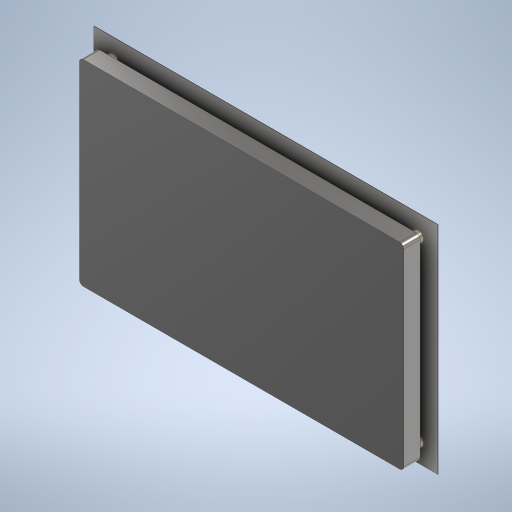
# Autodesk Inventor part: monitor-stand
Saved by Autodesk Inventor 2023 (Build 270158030, 158C)
## iProperties
Created: 2024-02-27
Part Number: monitor-stand
Material: Generic
Document SubType Name: Modeling
Designer: Imogen Heard
Density: 1 g/cm^3
Appearance: Expanded Metal 01
Author: Imogen Heard
Autodesk Inventor part; units mm, degrees
ref_plane "YZ Plane" through (0, 0, 0) normal (1, 0, 0) x (0, 1, 0)
ref_plane "XZ Plane" through (0, 0, 0) normal (0, 1, 0) x (-1, 0, 0)
ref_plane "XY Plane" through (0, 0, 0) normal (0, 0, 1) x (1, 0, 0)
sketch "Sketch1" plane through (0, 0, 0) normal (0, 0, 1) x (1, 0, 0)
  line L0 (-82.5, 50) -> (82.5, 50)
  line L1 (82.5, 50) -> (82.5, -50)
  line L2 (82.5, -50) -> (-82.5, -50)
  line L3 (-82.5, -50) -> (-82.5, 50)
  point P0 (0, 0)
  dimension "d0" = 165
  dimension "d1" = 100
  dimension "d2" = 82.5
  dimension "d3" = 50
  constraints: 8 end point, 2 parallel, 1 horizontal, 1 perpendicular
  measures "d0" distance between parallel lines of L1 L3
  measures "d1" distance between parallel lines of L2 L0
  measures "d2" horizontal distance of L2.end point (0, 0)
  measures "d3" distance from line of L2 point (0, 0)
extrude "Extrusion1" add sketch "Sketch1" along normal blind 8.36
sketch "Sketch2" plane through (0, 0, 0) normal (0, 0, -1) x (-1, 0, 0)
  circle A0 centre (-77.5, 45) radius 2.75
  circle A1 centre (77.5, 45) radius 2.75
  circle A2 centre (77.5, -45) radius 2.75
  circle A3 centre (-77.5, -45) radius 2.75
  line L0 (-82.5, 50) -> (82.5, 50) projected
  line L1 (-82.5, -50) -> (-82.5, 50) projected
  line L2 (82.5, -50) -> (-82.5, -50) projected
  line L3 (82.5, 50) -> (82.5, -50) projected
  point P0 (0, 0)
  dimension "d6" = 5.5
  dimension "d7" = 5
  dimension "d8" = 5
  dimension "d9" = 5
  dimension "d10" = 5
  constraints: 4 centre point, 3 equal radius, 2 horizontal alignment, 2 vertical alignment
  measures "d6" diameter of A3
  measures "d7" distance from line of L0 A0.centre
  measures "d8" distance from line of L1 A0.centre
  measures "d9" distance from line of L2 A3.centre
  measures "d10" distance from line of L3 A2.centre
extrude "Extrusion2" add sketch "Sketch2" along normal blind 4 contours A0 | A1 | A2 | A3
hole "Hole1" at (-77.5, -45, -4) direction (0, 0, 1) diameter 2.013 depth 4 tip angle 118 start extended yes countersink diameter 4 countersink angle 90 thread size "M2.5x0.45" class "6H" standard "ISO Metric profile"
hole "Hole2" at (77.5, 45, -4) direction (0, 0, 1) diameter 2.013 depth 4 tip angle 118 start extended yes countersink diameter 4 countersink angle 90 thread size "M2.5x0.45" class "6H" standard "ISO Metric profile"
hole "Hole3" at (77.5, -45, -4) direction (0, 0, 1) diameter 2.013 depth 4 tip angle 118 start extended yes countersink diameter 4 countersink angle 90 thread size "M2.5x0.45" class "6H" standard "ISO Metric profile"
hole "Hole4" at (-77.5, 45, -4) direction (0, 0, 1) diameter 2.013 depth 4 tip angle 118 start extended yes countersink diameter 4 countersink angle 90 thread size "M2.5x0.45" class "6H" standard "ISO Metric profile"
fillet "Fillet1" radius 2 4 edges at (82.5, 50, 4.18) (-82.5, 50, 4.18) (82.5, -50, 4.18) (-82.5, -50, 4.18)
sketch "Sketch4" plane through (0, 0, 0) normal (0, 0, -1) x (-1, 0, 0)
  line L0 (81.5, 35) -> (73.35, 35)
  line L1 (73.35, 35) -> (73.35, 23)
  line L2 (73.35, 23) -> (81.5, 23)
  line L3 (81.5, 23) -> (81.5, 35)
  line L4 (-80.5, 50) -> (80.5, 50) projected
  line L5 (82.5, 48) -> (82.5, -48) projected
  point P0 (0, 0)
  dimension "d54" = 15
  dimension "d55" = 12
  dimension "d56" = 9.15
  dimension "d57" = 1
  constraints: 8 end point, 2 parallel, 1 horizontal, 1 perpendicular
  measures "d54" distance between parallel lines of L0 L4
  measures "d55" distance between parallel lines of L2 L0
  measures "d56" distance between parallel lines of L5 L1
  measures "d57" distance between parallel lines of L5 L3
extrude "Extrusion3" add sketch "Sketch4" along normal blind 3
fillet "Fillet2" radius 6 2 edges at (-81.5, 35, -1.5) (-81.5, 23, -1.5)
sketch "Sketch5" plane through (0, 0, 0) normal (0, 0, -1) x (-1, 0, 0)
  arc A0 (77.425, 21.5) -> (77.425, 36.5) centre (77.425, 29) ccw
  line L0 (73.35, 35) -> (73.35, 23) projected
  line L1 (73.35, 23) -> (75.5, 23) projected
  line L2 (75.5, 35) -> (73.35, 35) projected
  line L3 (81.5, 35) -> (73.35, 35) projected
  line L4 (77.425, 36.5) -> (77.425, 21.5)
  arc A1 (75.5, 23) -> (75.5, 35) centre (75.5, 29) ccw projected
  point P0 (0, 0)
  point P1 (77.425, 35)
  point P2 (77.425, 35)
  point P3 (77.425, 23)
  point P4 (77.425, 34.6828)
  point P5 (77.425, 23.3172)
  point P6 (77.425, 35)
  dimension "d60" = 15
  dimension "d61" = 12
  dimension "d62" = 6
  dimension "d64" = 4.075
  constraints: 2 end point, 2 point on circle, 1 centre point, 1 midpoint
  measures "d60" diameter of A0
  measures "d61" distance from line of point (77.425, 35) L1
  measures "d62" distance from line of L1 A0.centre
  measures "d64" distance from line of L0 A0.centre
extrude "Extrusion4" add sketch "Sketch5" along normal blind 2.7 contours L4 A1 A0 | L4 A1
sketch "Sketch6" plane through (-82.5, -48, 8.36) normal (-1, 0, 0) x (0, 0, 1)
  line L0 (-14.66, 18.5) -> (-10.47, 18.5)
  line L1 (-10.47, 33.5) -> (-14.66, 33.5)
  line L2 (-14.66, 33.5) -> (-14.66, 18.5)
  line L3 (-10.47, 20) -> (-9.06, 21)
  line L4 (-9.06, 21) -> (-9.06, 31)
  line L5 (-8.36, 0) -> (-8.36, 96) projected
  line L6 (-9.06, 31) -> (-10.47, 32)
  line L7 (-10.47, 33) -> (-8.36, 33)
  line L8 (-8.36, 33) -> (-8.36, 33.5)
  line L9 (-8.36, 33.5) -> (-10.47, 33.5)
  line L10 (-10.47, 18.5) -> (-8.36, 18.5)
  line L11 (-8.36, 18.5) -> (-8.36, 19)
  line L12 (-8.36, 19) -> (-10.47, 19)
  line L13 (-8.36, -2) -> (0, -2) projected
  line L14 (-10.47, 19) -> (-10.47, 20)
  line L15 (-10.47, 32) -> (-10.47, 33)
  line L16 (-10.92, 33.05) -> (-10.92, 31.7675)
  line L17 (-10.92, 31.7675) -> (-9.51, 30.7675)
  line L18 (-9.51, 30.7675) -> (-9.51, 21.2325)
  line L19 (-9.51, 21.2325) -> (-10.92, 20.2325)
  line L20 (-10.92, 20.2325) -> (-10.92, 18.95)
  line L21 (-10.92, 18.95) -> (-14.21, 18.95)
  line L22 (-14.21, 18.95) -> (-14.21, 33.05)
  line L23 (-14.21, 33.05) -> (-10.92, 33.05)
  point P0 (-8.36, 48)
  point P1 (-12.565, 33.05)
  point P2 (-10.47, 32.5)
  point P3 (-10.47, 19.5)
  point P4 (-8.36, 18.5)
  point P5 (-10.47, 33.5)
  dimension "d68" = 0.5
  dimension "d69" = 0.5
  dimension "d70" = 15
  dimension "d71" = 6.3
  dimension "d73" = 0.7
  dimension "d74" = 1.5
  dimension "d75" = 1.5
  dimension "d76" = 20.5
  dimension "d77" = 2.5
  dimension "d78" = 2.5
  dimension "d79" = 2.11
  dimension "d80" = 0.45
  dimension "d81" = 0.45
  dimension "d82" = 0.45
  dimension "d83" = 0.45
  dimension "d84" = 0.45
  dimension "d85" = 0.45
  constraints: 44 end point, 9 parallel, 6 perpendicular, 3 horizontal, 3 midpoint, 2 point on line, 1 coincident, 1 vertical alignment, 2 other
  measures "d68" distance between parallel lines of L9 L7
  measures "d69" distance between parallel lines of L12 L10
  measures "d70" distance between parallel lines of L1 L0
  measures "d71" distance between parallel lines of L5 L2
  measures "d73" distance between parallel lines of L5 L4
  measures "d74" distance from line of L1 L6.end
  measures "d75" distance from line of L0 L3.start
  measures "d76" distance between parallel lines of L13 L0
  measures "d77" distance from line of L1 L4.end
  measures "d78" distance from line of L0 L3.end
  measures "d79" distance between parallel lines of L5 L15
  measures "d80" distance between parallel lines of L2 L22
  measures "d81" distance from line of L1 point (-12.565, 33.05)
  measures "d82" distance between parallel lines of L4 L18
  measures "d83" distance from line of point (-10.47, 32.5) L16
  measures "d84" distance between parallel lines of L0 L21
  measures "d85" distance from line of point (-10.47, 19.5) L20
extrude "Extrusion5" add sketch "Sketch6" along normal blind 0.4 and the other way blind 12 contours L2 L1 L9 L5 L7 L15 L6 L4 L3 L14 L12 L10 L0
fillet "Fillet3" radius 0.5 6 edges at (-76.7, -14.5, -6.3) (-76.7, -29.5, -6.3) (-76.7, -27.7675, -2.56) (-76.7, -16.2325, -2.56) (-76.7, -17, -0.7) (-76.7, -27, -0.7)
fillet "Fillet4" radius 0.2 8 edges at (-76.7, -29.05, -5.85) (-76.7, -14.95, -5.85) (-76.7, -29.05, -2.56) (-76.7, -26.7675, -1.15) (-76.7, -17.2325, -1.15) (-76.7, -14.95, -2.56) (-76.7, -16, -2.11) (-76.7, -28, -2.11)
sketch "Sketch7" plane through (-70.5, -48, 8.36) normal (-1, 0, 0) x (0, 0, -1)
  arc A0 (9.2708, -20.8505) -> (9.06, -21.2584) centre (9.56, -21.2584) ccw projected
  line L0 (10.3857, -20.0598) -> (9.2708, -20.8505) projected
  arc A1 (10.3857, -20.0598) -> (10.47, -19.8967) centre (10.27, -19.8967) ccw projected
  line L1 (10.47, -19) -> (10.47, -19.8967) projected
  line L2 (8.36, -19) -> (10.47, -19) projected
  line L3 (14.16, -18.5) -> (8.36, -18.5) projected
  arc A2 (14.66, -19) -> (14.16, -18.5) centre (14.16, -19) ccw projected
  line L4 (14.66, -33) -> (14.66, -19) projected
  arc A3 (14.16, -33.5) -> (14.66, -33) centre (14.16, -33) ccw projected
  line L5 (8.36, -33.5) -> (14.16, -33.5) projected
  line L6 (10.47, -33) -> (8.36, -33) projected
  line L7 (10.47, -32.1033) -> (10.47, -33) projected
  arc A4 (10.47, -32.1033) -> (10.3857, -31.9402) centre (10.27, -32.1033) ccw projected
  line L8 (9.2708, -31.1495) -> (10.3857, -31.9402) projected
  arc A5 (9.06, -30.7416) -> (9.2708, -31.1495) centre (9.56, -30.7416) ccw projected
  line L9 (9.06, -21.2584) -> (9.06, -30.7416) projected
  arc A6 (10.92, -32.0258) -> (10.7092, -31.618) centre (10.42, -32.0258) ccw projected
  line L10 (10.92, -32.85) -> (10.92, -32.0258) projected
  arc A7 (10.92, -32.85) -> (11.12, -33.05) centre (11.12, -32.85) ccw projected
  line L11 (14.01, -33.05) -> (11.12, -33.05) projected
  arc A8 (14.01, -33.05) -> (14.21, -32.85) centre (14.01, -32.85) ccw projected
  line L12 (14.21, -19.15) -> (14.21, -32.85) projected
  arc A9 (14.21, -19.15) -> (14.01, -18.95) centre (14.01, -19.15) ccw projected
  line L13 (11.12, -18.95) -> (14.01, -18.95) projected
  arc A10 (11.12, -18.95) -> (10.92, -19.15) centre (11.12, -19.15) ccw projected
  line L14 (10.92, -19.9742) -> (10.92, -19.15) projected
  arc A11 (10.7092, -20.382) -> (10.92, -19.9742) centre (10.42, -19.9742) ccw projected
  line L15 (9.5943, -21.1727) -> (10.7092, -20.382) projected
  arc A12 (9.5943, -21.1727) -> (9.51, -21.3359) centre (9.71, -21.3359) ccw projected
  line L16 (9.51, -30.6641) -> (9.51, -21.3359) projected
  arc A13 (9.51, -30.6641) -> (9.5943, -30.8273) centre (9.71, -30.6641) ccw projected
  line L17 (10.7092, -31.618) -> (9.5943, -30.8273) projected
  line L18 (8.36, -33) -> (8.36, -33.5) projected
  line L19 (8.36, -18.5) -> (8.36, -19) projected
  point P0 (8.36, -48)
extrude "Extrusion6" add sketch "Sketch7" along normal blind 4.5 contours A6 L17 A13 L16 A12 L15 A11 L14 A10 L13 A9 L12 A8 L11 A7 L10
sketch "Sketch8" plane through (-82.5, -48, 8.36) normal (-1, 0, 0) x (0, 0, 1)
  line L0 (-10.06, 42.6) -> (-10.06, 48.5) construction
  line L1 (-8.46, 42.6) -> (-8.46, 48.5)
  line L2 (-11.66, 48.5) -> (-11.66, 42.6)
  arc A0 (-11.66, 42.6) -> (-8.46, 42.6) centre (-10.06, 42.6) ccw
  arc A1 (-8.46, 48.5) -> (-11.66, 48.5) centre (-10.06, 48.5) ccw
  line L3 (-8.36, 71.4778) -> (-8.36, 33.5) projected
  line L4 (-11.31, 42.6) -> (-11.31, 48.5)
  arc A2 (-8.81, 48.5) -> (-11.31, 48.5) centre (-10.06, 48.5) ccw
  line L5 (-8.81, 48.5) -> (-8.81, 42.6)
  arc A3 (-11.31, 42.6) -> (-8.81, 42.6) centre (-10.06, 42.6) ccw
  point P0 (-8.36, 48)
  point P1 (-10.06, 45.55)
  point P2 (-10.06, 50.1)
  point P3 (-10.06, 41)
  point P4 (-8.36, -2)
  dimension "d94" = 9.1
  dimension "d95" = 3.2
  dimension "d96" = 0.1
  dimension "d97" = 43
  dimension "d98" = 0.35
  constraints: 12 end point, 10 point on circle, 4 centre point, 4 tangent, 2 parallel, 1 midpoint, 1 vertical, 3 other
  measures "d94" distance of point (-10.06, 50.1) point (-10.06, 41)
  measures "d95" distance between parallel lines of L1 L2
  measures "d96" distance between parallel lines of L3 L1
  measures "d97" vertical distance of point (-8.36, -2) point (-10.06, 41)
  measures "d98" distance between parallel lines of L2 L4
extrude "Extrusion7" add sketch "Sketch8" against normal blind 7.5
sketch "Sketch9" plane through (-75, -48, 8.36) normal (1, 0, 0) x (0, 0, -1)
  arc A0 (11.66, 48.5) -> (8.46, 48.5) centre (10.06, 48.5) ccw projected
  line L0 (8.46, 48.5) -> (8.46, 42.6) projected
  arc A1 (8.46, 42.6) -> (11.66, 42.6) centre (10.06, 42.6) ccw projected
  line L1 (11.66, 42.6) -> (11.66, 48.5) projected
  line L2 (8.81, 42.6) -> (8.81, 48.5) projected
  arc A2 (11.31, 48.5) -> (8.81, 48.5) centre (10.06, 48.5) ccw projected
  line L3 (11.31, 48.5) -> (11.31, 42.6) projected
  arc A3 (8.81, 42.6) -> (11.31, 42.6) centre (10.06, 42.6) ccw projected
  point P0 (8.36, 48)
extrude "Extrusion8" add sketch "Sketch9" against normal blind 2 contours L2 A2 L3 A3
sketch "Sketch10" plane through (-82.5, -48, 8.36) normal (-1, 0, 0) x (0, 0, 1)
  circle A0 centre (-10.91, 59) radius 2.45
  circle A1 centre (-10.91, 59) radius 1.72
  line L0 (-8.36, 71.4778) -> (-8.36, 33.5) projected
  line L1 (0, 98) -> (-8.36, 98) projected
  point P0 (-8.36, 48)
  dimension "d103" = 4.9
  dimension "d104" = 0.73
  dimension "d105" = 2.55
  dimension "d106" = 39
  constraints: 2 centre point, 1 concentric
  measures "d103" diameter of A0
  measures "d104" radial gap between concentric circles of A0 A1
  measures "d105" distance from line of L0 A0.centre
  measures "d106" distance from line of L1 A0.centre
extrude "Extrusion9" add sketch "Sketch10" against normal blind 14
sketch "Sketch11" plane through (-68.5, 11, -2.55) normal (1, 0, 0) x (0, 0, -1)
  line L0 (-2.55, 12.4778) -> (-2.55, -25.5) projected
  line L1 (2.45, 3.175) -> (-2.55, 3.175)
  line L2 (-2.55, 3.175) -> (-2.55, -3.175)
  line L3 (-2.55, -3.175) -> (2.45, -3.175)
  line L4 (2.45, -3.175) -> (2.45, 3.175)
  circle A0 centre (0, 0) radius 1.72 projected
  point P0 (-2.55, -11)
  point P1 (-2.55, 3.175)
  dimension "d109" = 6.35
  dimension "d110" = 3.175
  dimension "d111" = 5
  constraints: 8 end point, 2 parallel, 1 horizontal, 1 perpendicular, 1 point on line
  measures "d109" distance between parallel lines of L3 L1
  measures "d110" distance from line of A0.centre L3
  measures "d111" distance between parallel lines of L0 L4
extrude "Extrusion10" add sketch "Sketch11" against normal blind 12
sketch "Sketch12" plane through (0, 0, 0) normal (0, 0, -1) x (-1, 0, 0)
  line L0 (-63.9, 42.33) -> (-25.9, 42.33)
  line L1 (-25.9, 42.33) -> (-25.9, 24.33)
  line L2 (-25.9, 24.33) -> (-63.9, 24.33)
  line L3 (-63.9, 24.33) -> (-63.9, 42.33)
  line L4 (22.83, 42.33) -> (60.83, 42.33)
  line L5 (60.83, 42.33) -> (60.83, 24.33)
  line L6 (60.83, 24.33) -> (22.83, 24.33)
  line L7 (22.83, 24.33) -> (22.83, 42.33)
  line L8 (-82.5, -48) -> (-82.5, 48) projected
  line L9 (-80.5, 50) -> (80.5, 50) projected
  line L10 (82.5, 48) -> (82.5, 34.5222) projected
  point P0 (0, 0)
  dimension "d114" = 38
  dimension "d115" = 18
  dimension "d116" = 38
  dimension "d117" = 18.6
  dimension "d118" = 7.67
  dimension "d119" = 21.67
  constraints: 16 end point, 4 parallel, 2 horizontal, 2 horizontal alignment, 2 perpendicular, 2 point on line
  measures "d114" distance between parallel lines of L1 L3
  measures "d115" distance between parallel lines of L2 L0
  measures "d116" distance between parallel lines of L5 L7
  measures "d117" distance between parallel lines of L8 L3
  measures "d118" distance between parallel lines of L9 L0
  measures "d119" distance between parallel lines of L5 L10
extrude "Extrusion11" add sketch "Sketch12" along normal blind 5.09
fillet "Fillet5" radius 3 8 edges at (63.9, 24.33, -2.545) (63.9, 42.33, -2.545) (25.9, 24.33, -2.545) (25.9, 42.33, -2.545) (-60.83, 42.33, -2.545) (-22.83, 42.33, -2.545) (-22.83, 24.33, -2.545) (-60.83, 24.33, -2.545)
fillet "Fillet6" radius 0.2 16 edges at (-23.7087, 41.4513, -5.09) (-22.83, 33.33, -5.09) (-23.7087, 25.2087, -5.09) (-41.83, 24.33, -5.09) (-59.9513, 25.2087, -5.09) (-60.83, 33.33, -5.09) (-59.9513, 41.4513, -5.09) (-41.83, 42.33, -5.09) (26.7787, 41.4513, -5.09) (44.9, 42.33, -5.09) (63.0213, 41.4513, -5.09) (63.9, 33.33, -5.09) (63.0213, 25.2087, -5.09) (44.9, 24.33, -5.09) (26.7787, 25.2087, -5.09) (25.9, 33.33, -5.09)
sketch "Sketch13" plane through (77.5, 45, -4) normal (0, 0, -1) x (-1, 0, 0)
  line L0 (-10, 10) -> (165, 10)
  line L1 (165, 10) -> (165, -100)
  line L2 (165, -100) -> (-10, -100)
  line L3 (-10, -100) -> (-10, 10)
  line L4 (-3, 5) -> (158, 5) projected
  line L5 (-5, -93) -> (-5, 3) projected
  line L6 (160, -21.5222) -> (160, -59.5) projected
  line L7 (158, -95) -> (-3, -95) projected
  line L8 (2, -2) -> (153, -2)
  line L9 (153, -2) -> (153, -88)
  line L10 (153, -88) -> (2, -88)
  line L11 (2, -88) -> (2, -2)
  point P0 (77.5, -45)
  point P1 (-10, -45)
  dimension "d124" = 5
  dimension "d125" = 5
  dimension "d126" = 5
  dimension "d127" = 5
  dimension "d128" = 12
  dimension "d129" = 12
  dimension "d130" = 12
  dimension "d131" = 12
  constraints: 16 end point, 4 parallel, 2 horizontal, 2 perpendicular, 1 midpoint
  measures "d124" distance between parallel lines of L0 L4
  measures "d125" distance between parallel lines of L3 L5
  measures "d126" distance between parallel lines of L1 L6
  measures "d127" distance between parallel lines of L7 L2
  measures "d128" distance between parallel lines of L8 L0
  measures "d129" distance from line of point (-10, -45) L11
  measures "d130" distance between parallel lines of L2 L10
  measures "d131" distance between parallel lines of L1 L9
extrude "Extrusion12" add sketch "Sketch13" along normal blind 0.2
equation "\"d2\" = 0.5 * d0"
equation "\"d3\" = 0.5 * d1"
equation "\"d64\" = 0.5 * d63"
equation "\"d110\" = 0.5 * d109"
equation "\"d116\" = d114"
equation "\"d63\" = 8.15"
body "Solid1"
